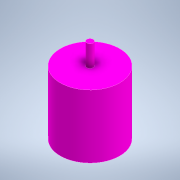
# Autodesk Inventor part: motor reaction wheel'
Saved by Autodesk Inventor 2021 (Build 250183000, 183)
## iProperties
Created: 2021-07-30
Part Number: motor reaction wheel'
Material: PVC, Unplasticized
Document SubType Name: Modeling
Designer: samlo
Density: 1.29 g/cm^3
Appearance: Magenta
Author: samlo
Autodesk Inventor part; units mm, degrees
ref_plane "YZ Plane" through (0, 0, 0) normal (1, 0, 0) x (0, 1, 0)
ref_plane "XZ Plane" through (0, 0, 0) normal (0, 1, 0) x (-1, 0, 0)
ref_plane "XY Plane" through (0, 0, 0) normal (0, 0, 1) x (1, 0, 0)
sketch "Sketch1" plane through (0, 0, 0) normal (0, 0, 1) x (1, 0, 0)
  line L0 (0, 0) -> (13.95, 0)
  line L1 (13.95, 0) -> (13.95, 29.7)
  line L2 (13.95, 29.7) -> (1.5, 29.7)
  line L3 (1.5, 29.7) -> (1.5, 39.7)
  line L4 (1.5, 39.7) -> (0, 39.7)
  line L5 (0, 39.7) -> (0, 0)
  dimension "d0" = 1.5
  dimension "d1" = 39.7
  dimension "d2" = 13.95
  dimension "d3" = 10
  constraints: 12 end point, 5 perpendicular, 1 horizontal
  measures "d0" distance of L3.end L4.end
  measures "d1" distance of L4.end L0.start
  measures "d2" distance of L0.start L0.end
  measures "d3" distance of L2.end L3.end
revolve "Revolution1" add sketch "Sketch1" angle 360 about axis through (0, 39.7, 0) along (0, -1, 0)
body "Solid1"
